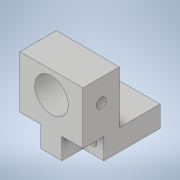
# Autodesk Inventor part: 00_micrometer_moun_xystage_china_new
Saved by Autodesk Inventor 2022 (Build 260153000, 153)
## iProperties
Created: 2021-05-08
Part Number: 00_micrometer_moun_xystage_china_new
Material: Generic
Document SubType Name: Modeling
Designer: diederichbenedict
Density: 1 g/cm^3
Appearance: Default
Author: diederichbenedict
Autodesk Inventor part; units mm, degrees
ref_plane "YZ Plane" through (0, 0, 0) normal (1, 0, 0) x (0, 1, 0)
ref_plane "XZ Plane" through (0, 0, 0) normal (0, 1, 0) x (-1, 0, 0)
ref_plane "XY Plane" through (0, 0, 0) normal (0, 0, 1) x (1, 0, 0)
sketch "Sketch1" plane through (0, 0, 0) normal (0, 0, 1) x (1, 0, 0)
  line L0 (0, 0) -> (-18, 0)
  line L1 (-18, 0) -> (-18, 6)
  line L2 (-18, 6) -> (0, 6)
  line L3 (0, 6) -> (0, 0)
  dimension "d0" = 18
  dimension "d1" = 6
  constraints: 8 end point, 2 parallel, 1 horizontal, 1 perpendicular
  measures "d0" distance of L1.end L2.end
  measures "d1" distance of L0.end L1.end
extrude "Extrusion1" add sketch "Sketch1" along normal blind 22
sketch "Sketch2" plane through (0, 0, 22) normal (0, 0, 1) x (1, 0, 0)
  line L0 (-18, 0) -> (0, 0) projected
  line L1 (0, 0) -> (0, 6) projected
  line L2 (0, 6) -> (-18, 6) projected
  line L3 (-18, 6) -> (-18, 0) projected
  circle A0 centre (-14.75, 3.2) radius 1.25
  circle A1 centre (-3.25, 3.2) radius 1.25
  dimension "d4" = 2.5
  dimension "d5" = 2.5
  dimension "d6" = 2.8
  dimension "d7" = 2.8
  dimension "d8" = 3.25
  dimension "d9" = 3.25
  dimension "d31" = 11.5
  constraints: 2 centre point
  measures "d4" diameter of A0
  measures "d5" diameter of A1
  measures "d6" distance from line of A0.centre L2
  measures "d7" distance from line of L2 A1.centre
  measures "d8" distance from line of A1.centre L1
  measures "d9" distance from line of A0.centre L3
  measures "d31" distance of A0.centre A1.centre
extrude "Extrusion2" cut sketch "Sketch2" against normal through all contours A0 | A1
sketch "Sketch3" plane through (0, 0, 0) normal (1, 0, 0) x (0, 0, -1)
  line L0 (0, 6) -> (0, 0) projected
  line L1 (0, 6) -> (-22, 6) projected
  line L2 (-22, 0) -> (-22, 6) projected
  line L3 (0, 0) -> (-22, 0) projected
  line L4 (0, 6) -> (-22, 6) projected
  line L5 (-22, 6) -> (-11.6, 6)
  line L6 (-11.6, 6) -> (-11.6, 21)
  line L7 (-11.6, 21) -> (-22, 21)
  line L8 (-22, 21) -> (-22, 6)
  dimension "d12" = 10.4
  dimension "d13" = 15
  constraints: 8 end point, 2 parallel, 1 horizontal, 1 perpendicular
  measures "d12" distance of L7.end L6.end
  measures "d13" distance of L6.end L5.end
extrude "Extrusion3" add sketch "Sketch3" against normal up to surface (18 mm away) contours L1 L8 L7 L6
sketch "Sketch4" plane through (0, 6, 11.6) normal (0, 0, -1) x (-1, 0, 0)
  line L0 (18, 0) -> (18, 15) projected
  line L1 (0, 15) -> (18, 15) projected
  line L2 (0, 15) -> (0, 0) projected
  line L3 (18, 0) -> (0, 0) projected
  circle A0 centre (9, 8.7) radius 4.8
  point P0 (0, -6)
  dimension "d16" = 9.6
  dimension "d17" = 6.3
  constraints: 1 centre point
  measures "d16" diameter of A0
  measures "d17" distance from line of A0.centre L1
extrude "Extrusion4" cut sketch "Sketch4" against normal through all contours A0
sketch "Sketch5" plane through (-18, 0, 0) normal (-1, 0, 0) x (0, 0, 1)
  line L0 (22.0213, 0) -> (16.0213, 0)
  line L1 (16.0213, 0) -> (16.0213, 6)
  line L2 (16.0213, 6) -> (22.0213, 6)
  line L3 (22.0213, 6) -> (22.0213, 0)
  point P0 (0, 0)
  dimension "d20" = 6
  dimension "d21" = 6
  constraints: 8 end point, 2 parallel, 1 horizontal, 1 perpendicular
  measures "d20" distance of L1.end L2.end
  measures "d21" distance of L0.end L1.end
extrude "Extrusion5" cut sketch "Sketch5" against normal blind 6
sketch "Sketch6" plane through (0, 0, 0) normal (1, 0, 0) x (0, 0, -1)
  line L0 (-22, 6) -> (-22, 0) projected
  line L1 (-16.0213, 6) -> (-22, 6) projected
  line L2 (-16.0213, 0) -> (-16.0213, 6) projected
  line L3 (-22, 0) -> (-16.0213, 0) projected
  point P0 (0, 0)
extrude "Extrusion6" cut sketch "Sketch6" against normal blind 6
sketch "Sketch7" plane through (0, 0, 0) normal (1, 0, 0) x (0, 0, -1)
  line L0 (-6.6, 12.2) -> (-11.6, 12.2)
  line L1 (-6.6, 17.2) -> (-11.6, 17.2)
  line L2 (-11.6, 21) -> (-11.6, 6) projected
  line L3 (-22, 6) -> (-22, 21) projected
  circle A0 centre (-16.8, 14.7) radius 1.4
  point P0 (0, 0)
  dimension "d26" = 2.8
  dimension "d27" = 5.2
  dimension "d28" = 2.5
  constraints: 4 end point, 2 horizontal, 1 centre point, 4 other
  measures "d26" diameter of A0
  measures "d27" distance from line of A0.centre L2
  measures "d28" distance from line of A0.centre L1
extrude "Extrusion7" cut sketch "Sketch7" against normal blind 6
equation "\"d9\" = d8"
body "Solid1"
